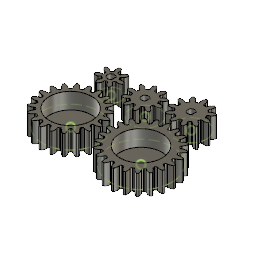
Telescope_Gears (Autodesk Fusion 360 design; units mm, degrees)
description: Spur Gear; Module: 2.0; Num Teeth: 20; Pressure Angle: 20.0; Backlash: 0.15 mm
description: Spur Gear; Module: 2.0; Num Teeth: 22; Pressure Angle: 20.0; Backlash: 0.15 mm
description: Spur Gear; Module: 2.0; Num Teeth: 11; Pressure Angle: 20.0; Backlash: 0.15 mm
description: Spur Gear; Module: 2.0; Num Teeth: 10; Pressure Angle: 20.0; Backlash: 0.15 mm
description: Spur Gear; Module: 2.0; Num Teeth: 7; Pressure Angle: 20.0; Backlash: 0.15 mm
Autodesk Fusion 360 part; units mm, degrees
(part 1 of 9)
sketch "Sketch1" plane through (0, 0, 0) normal (0, 0, 1) x (1, 0, 0) in component "Spur Gear (20 teeth) (1)"
  circle A0 centre (0, 0) radius 17.5492
  circle A1 centre (0, 0) radius 15
extrude "Extrude1" add sketch "Sketch1" along normal blind 11.5 makes body 1 in component "Spur Gear (20 teeth) (1)"
sketch "Sketch2" plane through (0, 0, 0) normal (0, 0, 1) x (1, 0, 0) in component "Spur Gear (20 teeth) (1)"
  spline S0 degree 5 poles (18.7151, -1.7185) (18.7245, -1.7194) (18.7433, -1.7209) (18.7715, -1.7223) (18.8091, -1.7228) (18.8563, -1.7215) (18.9035, -1.7188) (18.9507, -1.7153) (18.998, -1.7112) (19.0453, -1.7069) (19.0926, -1.7022) (19.1399, -1.697) (19.1872, -1.6913) (19.2346, -1.6849) (19.2819, -1.6778) (19.3293, -1.6701) (19.3766, -1.6618) (19.424, -1.6531) (19.4713, -1.644) (19.5186, -1.6345) (19.566, -1.6246) (19.6133, -1.6144) (19.6606, -1.6037) (19.7079, -1.5926) (19.7552, -1.581) (19.8025, -1.5691) (19.8498, -1.5568) (19.897, -1.5441) (19.9443, -1.531) (19.9915, -1.5176) (20.0387, -1.5039) (20.0858, -1.4898) (20.133, -1.4754) (20.1801, -1.4606) (20.2272, -1.4455) (20.2743, -1.43) (20.3213, -1.4143) (20.3683, -1.3982) (20.4153, -1.3818) (20.4623, -1.365) (20.5092, -1.348) (20.5561, -1.3307) (20.603, -1.313) (20.6498, -1.2951) (20.6966, -1.2768) (20.7434, -1.2583) (20.7901, -1.2394) (20.8368, -1.2203) (20.8835, -1.2009) (20.9301, -1.1812) (20.9767, -1.1612) (21.0233, -1.1409) (21.0698, -1.1204) (21.1162, -1.0995) (21.1627, -1.0784) (21.209, -1.0571) (21.2554, -1.0354) (21.3017, -1.0135) (21.3479, -0.9913) (21.3941, -0.9689) (21.4403, -0.9462) (21.4864, -0.9232) (21.5324, -0.8999) (21.5785, -0.8764) (21.6244, -0.8527) (21.6703, -0.8287) (21.7162, -0.8044) (21.762, -0.7799) (21.8078, -0.7551) (21.8535, -0.7301) (21.8991, -0.7049) (21.9356, -0.6845) (21.963, -0.669) (21.9812, -0.6587) (21.9903, -0.6535) knots 0 0 0 0 0 0 0.01428571 0.02857143 0.04285714 0.05714286 0.07142857 0.08571429 0.1 0.11428571 0.12857143 0.14285714 0.15714286 0.17142857 0.18571429 0.2 0.21428571 0.22857143 0.24285714 0.25714286 0.27142857 0.28571429 0.3 0.31428571 0.32857143 0.34285714 0.35714286 0.37142857 0.38571429 0.4 0.41428571 0.42857143 0.44285714 0.45714286 0.47142857 0.48571429 0.5 0.51428571 0.52857143 0.54285714 0.55714286 0.57142857 0.58571429 0.6 0.61428571 0.62857143 0.64285714 0.65714286 0.67142857 0.68571429 0.7 0.71428571 0.72857143 0.74285714 0.75714286 0.77142857 0.78571429 0.8 0.81428571 0.82857143 0.84285714 0.85714286 0.87142857 0.88571429 0.9 0.91428571 0.92857143 0.94285714 0.95714286 0.97142857 0.98571429 1 1 1 1 1 1
  spline S1 degree 5 poles (18.7151, 1.7185) (18.7245, 1.7194) (18.7433, 1.7209) (18.7715, 1.7223) (18.8091, 1.7228) (18.8563, 1.7215) (18.9035, 1.7188) (18.9507, 1.7153) (18.998, 1.7112) (19.0453, 1.7069) (19.0926, 1.7022) (19.1399, 1.697) (19.1872, 1.6913) (19.2346, 1.6849) (19.2819, 1.6778) (19.3293, 1.6701) (19.3766, 1.6618) (19.424, 1.6531) (19.4713, 1.644) (19.5186, 1.6345) (19.566, 1.6246) (19.6133, 1.6144) (19.6606, 1.6037) (19.7079, 1.5926) (19.7552, 1.581) (19.8025, 1.5691) (19.8498, 1.5568) (19.897, 1.5441) (19.9443, 1.531) (19.9915, 1.5176) (20.0387, 1.5039) (20.0858, 1.4898) (20.133, 1.4754) (20.1801, 1.4606) (20.2272, 1.4455) (20.2743, 1.43) (20.3213, 1.4143) (20.3683, 1.3982) (20.4153, 1.3818) (20.4623, 1.365) (20.5092, 1.348) (20.5561, 1.3307) (20.603, 1.313) (20.6498, 1.2951) (20.6966, 1.2768) (20.7434, 1.2583) (20.7901, 1.2394) (20.8368, 1.2203) (20.8835, 1.2009) (20.9301, 1.1812) (20.9767, 1.1612) (21.0233, 1.1409) (21.0698, 1.1204) (21.1162, 1.0995) (21.1627, 1.0784) (21.209, 1.0571) (21.2554, 1.0354) (21.3017, 1.0135) (21.3479, 0.9913) (21.3941, 0.9689) (21.4403, 0.9462) (21.4864, 0.9232) (21.5324, 0.8999) (21.5785, 0.8764) (21.6244, 0.8527) (21.6703, 0.8287) (21.7162, 0.8044) (21.762, 0.7799) (21.8078, 0.7551) (21.8535, 0.7301) (21.8991, 0.7049) (21.9356, 0.6845) (21.963, 0.669) (21.9812, 0.6587) (21.9903, 0.6535) knots 0 0 0 0 0 0 0.01428571 0.02857143 0.04285714 0.05714286 0.07142857 0.08571429 0.1 0.11428571 0.12857143 0.14285714 0.15714286 0.17142857 0.18571429 0.2 0.21428571 0.22857143 0.24285714 0.25714286 0.27142857 0.28571429 0.3 0.31428571 0.32857143 0.34285714 0.35714286 0.37142857 0.38571429 0.4 0.41428571 0.42857143 0.44285714 0.45714286 0.47142857 0.48571429 0.5 0.51428571 0.52857143 0.54285714 0.55714286 0.57142857 0.58571429 0.6 0.61428571 0.62857143 0.64285714 0.65714286 0.67142857 0.68571429 0.7 0.71428571 0.72857143 0.74285714 0.75714286 0.77142857 0.78571429 0.8 0.81428571 0.82857143 0.84285714 0.85714286 0.87142857 0.88571429 0.9 0.91428571 0.92857143 0.94285714 0.95714286 0.97142857 0.98571429 1 1 1 1 1 1
  arc A0 (21.9903, -0.6535) -> (21.9903, 0.6535) centre (0, 0) ccw
  line L0 (17.4657, -1.6047) -> (18.7151, -1.7185)
  line L1 (17.4657, 1.6047) -> (18.7151, 1.7185)
  line L2 (17.4657, -1.6047) -> (17.4657, 1.6047)
  point P0 (18.9453, -1.7156)
  point P1 (19.1773, -1.6924)
  point P2 (19.4104, -1.6555)
  point P3 (19.6442, -1.6073)
  point P4 (19.8786, -1.549)
  point P5 (20.1134, -1.4813)
  point P6 (20.3485, -1.4049)
  point P7 (20.5836, -1.3203)
  point P8 (20.8188, -1.2277)
  point P9 (21.0538, -1.1274)
  point P10 (21.2886, -1.0197)
  point P11 (21.523, -0.9047)
  point P12 (21.7569, -0.7826)
  point P13 (18.9453, 1.7156)
  point P14 (19.1773, 1.6924)
  point P15 (19.4104, 1.6555)
  point P16 (19.6442, 1.6073)
  point P17 (19.8786, 1.549)
  point P18 (20.1134, 1.4813)
  point P19 (20.3485, 1.4049)
  point P20 (20.5836, 1.3203)
  point P21 (20.8188, 1.2277)
  point P22 (21.0538, 1.1274)
  point P23 (21.2886, 1.0197)
  point P24 (21.523, 0.9047)
  point P25 (21.7569, 0.7826)
extrude "Extrude2" add sketch "Sketch2" along normal blind 11.5 bodies 1 in component "Spur Gear (20 teeth) (1)"
fillet "Fillet1" radius 0.9 2 edges at (17.4756, -1.6056, 5.75) (17.4756, 1.6056, 5.75) on bodies 1 in component "Spur Gear (20 teeth) (1)"
pattern_circular "C-Pattern1" count 20 over 360 about axis through (0, 0, 0) along (0, 0, 1) of "Extrude2", "Fillet1" in component "Spur Gear (20 teeth) (1)"
sketch "Sketch3" plane through (0, 0, 0) normal (0, 0, 1) x (1, 0, 0) in component "Spur Gear (20 teeth) (1)"
  circle A0 centre (0, 0) radius 20 construction
sketch "Sketch1 (2)" plane through (0, 0, 0) normal (0, 0, 1) x (1, 0, 0) in component "Spur Gear (22 teeth)"
  circle A0 centre (0, 0) radius 19.5492
  circle A1 centre (0, 0) radius 15
extrude "Extrude1'" add sketch "Sketch1 (2)" along normal blind 11.5 separate body makes body 2 in component "Spur Gear (22 teeth)"
sketch "Sketch2 (2)" plane through (0, 0, 0) normal (0, 0, 1) x (1, 0, 0) in component "Spur Gear (22 teeth)"
  spline S0 degree 5 poles (20.5993, -1.7469) (20.609, -1.7477) (20.6285, -1.7491) (20.6577, -1.7504) (20.6968, -1.7508) (20.7456, -1.7493) (20.7945, -1.7463) (20.8434, -1.7425) (20.8924, -1.7383) (20.9414, -1.7337) (20.9903, -1.7287) (21.0393, -1.7234) (21.0884, -1.7174) (21.1374, -1.7107) (21.1864, -1.7034) (21.2354, -1.6955) (21.2844, -1.6869) (21.3334, -1.678) (21.3825, -1.6686) (21.4315, -1.6589) (21.4805, -1.6487) (21.5294, -1.6382) (21.5784, -1.6273) (21.6274, -1.6159) (21.6763, -1.6041) (21.7253, -1.5919) (21.7742, -1.5794) (21.8231, -1.5664) (21.872, -1.5531) (21.9208, -1.5395) (21.9696, -1.5255) (22.0185, -1.5111) (22.0673, -1.4965) (22.116, -1.4814) (22.1648, -1.4661) (22.2135, -1.4504) (22.2622, -1.4343) (22.3109, -1.418) (22.3595, -1.4013) (22.4081, -1.3843) (22.4567, -1.3671) (22.5052, -1.3495) (22.5537, -1.3316) (22.6022, -1.3134) (22.6507, -1.2949) (22.6991, -1.2761) (22.7475, -1.257) (22.7958, -1.2376) (22.8441, -1.218) (22.8924, -1.198) (22.9406, -1.1778) (22.9888, -1.1573) (23.037, -1.1365) (23.0851, -1.1154) (23.1332, -1.0941) (23.1812, -1.0724) (23.2292, -1.0506) (23.2772, -1.0284) (23.3251, -1.006) (23.3729, -0.9833) (23.4207, -0.9604) (23.4685, -0.9372) (23.5162, -0.9137) (23.5639, -0.89) (23.6115, -0.866) (23.6591, -0.8417) (23.7067, -0.8173) (23.7541, -0.7925) (23.8016, -0.7675) (23.849, -0.7423) (23.8963, -0.7168) (23.9341, -0.6962) (23.9625, -0.6807) (23.9813, -0.6702) (23.9908, -0.665) knots 0 0 0 0 0 0 0.01428571 0.02857143 0.04285714 0.05714286 0.07142857 0.08571429 0.1 0.11428571 0.12857143 0.14285714 0.15714286 0.17142857 0.18571429 0.2 0.21428571 0.22857143 0.24285714 0.25714286 0.27142857 0.28571429 0.3 0.31428571 0.32857143 0.34285714 0.35714286 0.37142857 0.38571429 0.4 0.41428571 0.42857143 0.44285714 0.45714286 0.47142857 0.48571429 0.5 0.51428571 0.52857143 0.54285714 0.55714286 0.57142857 0.58571429 0.6 0.61428571 0.62857143 0.64285714 0.65714286 0.67142857 0.68571429 0.7 0.71428571 0.72857143 0.74285714 0.75714286 0.77142857 0.78571429 0.8 0.81428571 0.82857143 0.84285714 0.85714286 0.87142857 0.88571429 0.9 0.91428571 0.92857143 0.94285714 0.95714286 0.97142857 0.98571429 1 1 1 1 1 1
  spline S1 degree 5 poles (20.5993, 1.7469) (20.609, 1.7477) (20.6285, 1.7491) (20.6577, 1.7504) (20.6968, 1.7508) (20.7456, 1.7493) (20.7945, 1.7463) (20.8434, 1.7425) (20.8924, 1.7383) (20.9414, 1.7337) (20.9903, 1.7287) (21.0393, 1.7234) (21.0884, 1.7174) (21.1374, 1.7107) (21.1864, 1.7034) (21.2354, 1.6955) (21.2844, 1.6869) (21.3334, 1.678) (21.3825, 1.6686) (21.4315, 1.6589) (21.4805, 1.6487) (21.5294, 1.6382) (21.5784, 1.6273) (21.6274, 1.6159) (21.6763, 1.6041) (21.7253, 1.5919) (21.7742, 1.5794) (21.8231, 1.5664) (21.872, 1.5531) (21.9208, 1.5395) (21.9696, 1.5255) (22.0185, 1.5111) (22.0673, 1.4965) (22.116, 1.4814) (22.1648, 1.4661) (22.2135, 1.4504) (22.2622, 1.4343) (22.3109, 1.418) (22.3595, 1.4013) (22.4081, 1.3843) (22.4567, 1.3671) (22.5052, 1.3495) (22.5537, 1.3316) (22.6022, 1.3134) (22.6507, 1.2949) (22.6991, 1.2761) (22.7475, 1.257) (22.7958, 1.2376) (22.8441, 1.218) (22.8924, 1.198) (22.9406, 1.1778) (22.9888, 1.1573) (23.037, 1.1365) (23.0851, 1.1154) (23.1332, 1.0941) (23.1812, 1.0724) (23.2292, 1.0506) (23.2772, 1.0284) (23.3251, 1.006) (23.3729, 0.9833) (23.4207, 0.9604) (23.4685, 0.9372) (23.5162, 0.9137) (23.5639, 0.89) (23.6115, 0.866) (23.6591, 0.8417) (23.7067, 0.8173) (23.7541, 0.7925) (23.8016, 0.7675) (23.849, 0.7423) (23.8963, 0.7168) (23.9341, 0.6962) (23.9625, 0.6807) (23.9813, 0.6702) (23.9908, 0.665) knots 0 0 0 0 0 0 0.01428571 0.02857143 0.04285714 0.05714286 0.07142857 0.08571429 0.1 0.11428571 0.12857143 0.14285714 0.15714286 0.17142857 0.18571429 0.2 0.21428571 0.22857143 0.24285714 0.25714286 0.27142857 0.28571429 0.3 0.31428571 0.32857143 0.34285714 0.35714286 0.37142857 0.38571429 0.4 0.41428571 0.42857143 0.44285714 0.45714286 0.47142857 0.48571429 0.5 0.51428571 0.52857143 0.54285714 0.55714286 0.57142857 0.58571429 0.6 0.61428571 0.62857143 0.64285714 0.65714286 0.67142857 0.68571429 0.7 0.71428571 0.72857143 0.74285714 0.75714286 0.77142857 0.78571429 0.8 0.81428571 0.82857143 0.84285714 0.85714286 0.87142857 0.88571429 0.9 0.91428571 0.92857143 0.94285714 0.95714286 0.97142857 0.98571429 1 1 1 1 1 1
  arc A0 (23.9908, -0.665) -> (23.9908, 0.665) centre (0, 0) ccw
  line L0 (19.4693, -1.6519) -> (20.5993, -1.7469)
  line L1 (19.4693, 1.6519) -> (20.5993, 1.7469)
  line L2 (19.4693, -1.6519) -> (19.4693, 1.6519)
  point P0 (20.8381, -1.7429)
  point P1 (21.0786, -1.7185)
  point P2 (21.32, -1.6804)
  point P3 (21.5622, -1.6309)
  point P4 (21.8048, -1.5712)
  point P5 (22.0479, -1.5022)
  point P6 (22.2911, -1.4246)
  point P7 (22.5345, -1.3386)
  point P8 (22.7779, -1.2448)
  point P9 (23.0211, -1.1433)
  point P10 (23.2641, -1.0344)
  point P11 (23.5068, -0.9183)
  point P12 (23.7491, -0.7951)
  point P13 (20.8381, 1.7429)
  point P14 (21.0786, 1.7185)
  point P15 (21.32, 1.6804)
  point P16 (21.5622, 1.6309)
  point P17 (21.8048, 1.5712)
  point P18 (22.0479, 1.5022)
  point P19 (22.2911, 1.4246)
  point P20 (22.5345, 1.3386)
  point P21 (22.7779, 1.2448)
  point P22 (23.0211, 1.1433)
  point P23 (23.2641, 1.0344)
  point P24 (23.5068, 0.9183)
  point P25 (23.7491, 0.7951)
extrude "Extrude2'" add sketch "Sketch2 (2)" along normal blind 11.5 bodies 2 in component "Spur Gear (22 teeth)"
fillet "Fillet1'" radius 1 2 edges at (19.4792, -1.6527, 5.75) (19.4792, 1.6527, 5.75) on bodies 2 in component "Spur Gear (22 teeth)"
pattern_circular "C-Pattern1'" count 22 over 360 about axis through (0, 0, 0) along (0, 0, 1) of "Extrude2'", "Fillet1'" in component "Spur Gear (22 teeth)"
sketch "Sketch3 (2)" plane through (0, 0, 0) normal (0, 0, 1) x (1, 0, 0) in component "Spur Gear (22 teeth)"
  circle A0 centre (0, 0) radius 22 construction
sketch "Sketch1 (3)" plane through (0, 0, 0) normal (0, 0, 1) x (1, 0, 0) in component "Spur Gear (11 teeth)"
  circle A0 centre (0, 0) radius 8.5492
  circle A1 centre (0, 0) radius 2.5
extrude "Extrude1''" add sketch "Sketch1 (3)" along normal blind 11.5 separate body makes body 3 in component "Spur Gear (11 teeth)"
sketch "Sketch2 (3)" plane through (0, 0, 0) normal (0, 0, 1) x (1, 0, 0) in component "Spur Gear (11 teeth)"
  spline S0 degree 5 poles (10.2138, -1.5886) (10.2216, -1.5898) (10.2373, -1.5919) (10.2609, -1.5944) (10.2925, -1.5962) (10.3321, -1.5965) (10.3719, -1.5954) (10.4117, -1.5933) (10.4517, -1.5907) (10.4917, -1.5878) (10.5317, -1.5846) (10.5717, -1.5809) (10.6118, -1.5765) (10.6519, -1.5714) (10.6921, -1.5656) (10.7323, -1.5592) (10.7726, -1.5521) (10.8128, -1.5446) (10.8531, -1.5367) (10.8933, -1.5283) (10.9336, -1.5196) (10.9739, -1.5104) (11.0141, -1.5007) (11.0544, -1.4906) (11.0947, -1.4801) (11.135, -1.4691) (11.1752, -1.4577) (11.2155, -1.4459) (11.2557, -1.4337) (11.2959, -1.4211) (11.3362, -1.4082) (11.3763, -1.3948) (11.4165, -1.3811) (11.4567, -1.367) (11.4968, -1.3526) (11.5369, -1.3378) (11.577, -1.3226) (11.617, -1.307) (11.657, -1.2912) (11.697, -1.2749) (11.7369, -1.2583) (11.7769, -1.2414) (11.8167, -1.2242) (11.8566, -1.2066) (11.8963, -1.1887) (11.9361, -1.1704) (11.9758, -1.1518) (12.0154, -1.1329) (12.0551, -1.1137) (12.0946, -1.0941) (12.1341, -1.0743) (12.1736, -1.0541) (12.213, -1.0336) (12.2524, -1.0128) (12.2916, -0.9917) (12.3309, -0.9703) (12.3701, -0.9486) (12.4092, -0.9265) (12.4482, -0.9042) (12.4872, -0.8816) (12.5262, -0.8587) (12.565, -0.8355) (12.6038, -0.812) (12.6426, -0.7882) (12.6812, -0.7641) (12.7198, -0.7397) (12.7584, -0.715) (12.7968, -0.6901) (12.8352, -0.6649) (12.8735, -0.6393) (12.9117, -0.6136) (12.9422, -0.5927) (12.9651, -0.5769) (12.9803, -0.5664) (12.9879, -0.5611) knots 0 0 0 0 0 0 0.01428571 0.02857143 0.04285714 0.05714286 0.07142857 0.08571429 0.1 0.11428571 0.12857143 0.14285714 0.15714286 0.17142857 0.18571429 0.2 0.21428571 0.22857143 0.24285714 0.25714286 0.27142857 0.28571429 0.3 0.31428571 0.32857143 0.34285714 0.35714286 0.37142857 0.38571429 0.4 0.41428571 0.42857143 0.44285714 0.45714286 0.47142857 0.48571429 0.5 0.51428571 0.52857143 0.54285714 0.55714286 0.57142857 0.58571429 0.6 0.61428571 0.62857143 0.64285714 0.65714286 0.67142857 0.68571429 0.7 0.71428571 0.72857143 0.74285714 0.75714286 0.77142857 0.78571429 0.8 0.81428571 0.82857143 0.84285714 0.85714286 0.87142857 0.88571429 0.9 0.91428571 0.92857143 0.94285714 0.95714286 0.97142857 0.98571429 1 1 1 1 1 1
  spline S1 degree 5 poles (10.2138, 1.5886) (10.2216, 1.5898) (10.2373, 1.5919) (10.2609, 1.5944) (10.2925, 1.5962) (10.3321, 1.5965) (10.3719, 1.5954) (10.4117, 1.5933) (10.4517, 1.5907) (10.4917, 1.5878) (10.5317, 1.5846) (10.5717, 1.5809) (10.6118, 1.5765) (10.6519, 1.5714) (10.6921, 1.5656) (10.7323, 1.5592) (10.7726, 1.5521) (10.8128, 1.5446) (10.8531, 1.5367) (10.8933, 1.5283) (10.9336, 1.5196) (10.9739, 1.5104) (11.0141, 1.5007) (11.0544, 1.4906) (11.0947, 1.4801) (11.135, 1.4691) (11.1752, 1.4577) (11.2155, 1.4459) (11.2557, 1.4337) (11.2959, 1.4211) (11.3362, 1.4082) (11.3763, 1.3948) (11.4165, 1.3811) (11.4567, 1.367) (11.4968, 1.3526) (11.5369, 1.3378) (11.577, 1.3226) (11.617, 1.307) (11.657, 1.2912) (11.697, 1.2749) (11.7369, 1.2583) (11.7769, 1.2414) (11.8167, 1.2242) (11.8566, 1.2066) (11.8963, 1.1887) (11.9361, 1.1704) (11.9758, 1.1518) (12.0154, 1.1329) (12.0551, 1.1137) (12.0946, 1.0941) (12.1341, 1.0743) (12.1736, 1.0541) (12.213, 1.0336) (12.2524, 1.0128) (12.2916, 0.9917) (12.3309, 0.9703) (12.3701, 0.9486) (12.4092, 0.9265) (12.4482, 0.9042) (12.4872, 0.8816) (12.5262, 0.8587) (12.565, 0.8355) (12.6038, 0.812) (12.6426, 0.7882) (12.6812, 0.7641) (12.7198, 0.7397) (12.7584, 0.715) (12.7968, 0.6901) (12.8352, 0.6649) (12.8735, 0.6393) (12.9117, 0.6136) (12.9422, 0.5927) (12.9651, 0.5769) (12.9803, 0.5664) (12.9879, 0.5611) knots 0 0 0 0 0 0 0.01428571 0.02857143 0.04285714 0.05714286 0.07142857 0.08571429 0.1 0.11428571 0.12857143 0.14285714 0.15714286 0.17142857 0.18571429 0.2 0.21428571 0.22857143 0.24285714 0.25714286 0.27142857 0.28571429 0.3 0.31428571 0.32857143 0.34285714 0.35714286 0.37142857 0.38571429 0.4 0.41428571 0.42857143 0.44285714 0.45714286 0.47142857 0.48571429 0.5 0.51428571 0.52857143 0.54285714 0.55714286 0.57142857 0.58571429 0.6 0.61428571 0.62857143 0.64285714 0.65714286 0.67142857 0.68571429 0.7 0.71428571 0.72857143 0.74285714 0.75714286 0.77142857 0.78571429 0.8 0.81428571 0.82857143 0.84285714 0.85714286 0.87142857 0.88571429 0.9 0.91428571 0.92857143 0.94285714 0.95714286 0.97142857 0.98571429 1 1 1 1 1 1
  arc A0 (12.9879, -0.5611) -> (12.9879, 0.5611) centre (0, 0) ccw
  line L0 (8.4378, -1.3139) -> (10.2138, -1.5886)
  line L1 (8.4378, 1.3139) -> (10.2138, 1.5886)
  line L2 (8.4378, -1.3139) -> (8.4378, 1.3139)
  point P0 (10.4056, -1.5935)
  point P1 (10.6003, -1.5776)
  point P2 (10.797, -1.5475)
  point P3 (10.995, -1.5052)
  point P4 (11.194, -1.4521)
  point P5 (11.3937, -1.3888)
  point P6 (11.5939, -1.316)
  point P7 (11.7942, -1.2339)
  point P8 (11.9945, -1.1429)
  point P9 (12.1945, -1.0432)
  point P10 (12.3941, -0.935)
  point P11 (12.5929, -0.8185)
  point P12 (12.791, -0.6938)
  point P13 (10.4056, 1.5935)
  point P14 (10.6003, 1.5776)
  point P15 (10.797, 1.5475)
  point P16 (10.995, 1.5052)
  point P17 (11.194, 1.4521)
  point P18 (11.3937, 1.3888)
  point P19 (11.5939, 1.316)
  point P20 (11.7942, 1.2339)
  point P21 (11.9945, 1.1429)
  point P22 (12.1945, 1.0432)
  point P23 (12.3941, 0.935)
  point P24 (12.5929, 0.8185)
  point P25 (12.791, 0.6938)
extrude "Extrude2''" add sketch "Sketch2 (3)" along normal blind 11.5 bodies 3 in component "Spur Gear (11 teeth)"
fillet "Fillet1''" radius 0.5 2 edges at (8.4474, -1.3154, 5.75) (8.4474, 1.3154, 5.75) on bodies 3 in component "Spur Gear (11 teeth)"
pattern_circular "C-Pattern1''" count 11 over 360 about axis through (0, 0, 0) along (0, 0, 1) of "Extrude2''", "Fillet1''" in component "Spur Gear (11 teeth)"
sketch "Sketch3 (3)" plane through (0, 0, 0) normal (0, 0, 1) x (1, 0, 0) in component "Spur Gear (11 teeth)"
  circle A0 centre (0, 0) radius 11 construction
sketch "Sketch1 (4)" plane through (0, 0, 0) normal (0, 0, 1) x (1, 0, 0) in component "Spur Gear (10 teeth)"
  circle A0 centre (0, 0) radius 7.5492
  circle A1 centre (0, 0) radius 2.5
extrude "Extrude1'''" add sketch "Sketch1 (4)" along normal blind 11.5 separate body makes body 4 in component "Spur Gear (10 teeth)"
sketch "Sketch2 (4)" plane through (0, 0, 0) normal (0, 0, 1) x (1, 0, 0) in component "Spur Gear (10 teeth)"
  spline S0 degree 5 poles (9.2643, -1.5734) (9.2719, -1.5747) (9.2872, -1.5771) (9.3103, -1.5797) (9.3412, -1.5819) (9.38, -1.5824) (9.419, -1.5816) (9.4582, -1.5798) (9.4973, -1.5775) (9.5366, -1.5749) (9.5758, -1.5719) (9.6151, -1.5684) (9.6545, -1.5643) (9.6939, -1.5594) (9.7333, -1.5538) (9.7728, -1.5475) (9.8124, -1.5407) (9.8519, -1.5333) (9.8915, -1.5255) (9.931, -1.5173) (9.9706, -1.5087) (10.0102, -1.4996) (10.0498, -1.4901) (10.0894, -1.4801) (10.129, -1.4697) (10.1686, -1.4587) (10.2082, -1.4474) (10.2477, -1.4356) (10.2873, -1.4235) (10.3269, -1.411) (10.3664, -1.398) (10.4059, -1.3847) (10.4454, -1.371) (10.4849, -1.3569) (10.5243, -1.3424) (10.5638, -1.3276) (10.6032, -1.3124) (10.6425, -1.2968) (10.6819, -1.2808) (10.7212, -1.2645) (10.7604, -1.2479) (10.7997, -1.2308) (10.8388, -1.2135) (10.878, -1.1958) (10.9171, -1.1777) (10.9561, -1.1593) (10.9952, -1.1406) (11.0341, -1.1215) (11.073, -1.1022) (11.1119, -1.0824) (11.1507, -1.0624) (11.1894, -1.042) (11.2281, -1.0213) (11.2668, -1.0003) (11.3054, -0.9789) (11.3439, -0.9573) (11.3823, -0.9353) (11.4207, -0.913) (11.459, -0.8905) (11.4973, -0.8676) (11.5355, -0.8443) (11.5736, -0.8208) (11.6116, -0.797) (11.6496, -0.7729) (11.6875, -0.7485) (11.7253, -0.7238) (11.763, -0.6988) (11.8007, -0.6735) (11.8383, -0.6479) (11.8758, -0.622) (11.9132, -0.5958) (11.943, -0.5746) (11.9654, -0.5586) (11.9803, -0.5479) (11.9877, -0.5425) knots 0 0 0 0 0 0 0.01428571 0.02857143 0.04285714 0.05714286 0.07142857 0.08571429 0.1 0.11428571 0.12857143 0.14285714 0.15714286 0.17142857 0.18571429 0.2 0.21428571 0.22857143 0.24285714 0.25714286 0.27142857 0.28571429 0.3 0.31428571 0.32857143 0.34285714 0.35714286 0.37142857 0.38571429 0.4 0.41428571 0.42857143 0.44285714 0.45714286 0.47142857 0.48571429 0.5 0.51428571 0.52857143 0.54285714 0.55714286 0.57142857 0.58571429 0.6 0.61428571 0.62857143 0.64285714 0.65714286 0.67142857 0.68571429 0.7 0.71428571 0.72857143 0.74285714 0.75714286 0.77142857 0.78571429 0.8 0.81428571 0.82857143 0.84285714 0.85714286 0.87142857 0.88571429 0.9 0.91428571 0.92857143 0.94285714 0.95714286 0.97142857 0.98571429 1 1 1 1 1 1
  spline S1 degree 5 poles (9.2643, 1.5734) (9.2719, 1.5747) (9.2872, 1.5771) (9.3103, 1.5797) (9.3412, 1.5819) (9.38, 1.5824) (9.419, 1.5816) (9.4582, 1.5798) (9.4973, 1.5775) (9.5366, 1.5749) (9.5758, 1.5719) (9.6151, 1.5684) (9.6545, 1.5643) (9.6939, 1.5594) (9.7333, 1.5538) (9.7728, 1.5475) (9.8124, 1.5407) (9.8519, 1.5333) (9.8915, 1.5255) (9.931, 1.5173) (9.9706, 1.5087) (10.0102, 1.4996) (10.0498, 1.4901) (10.0894, 1.4801) (10.129, 1.4697) (10.1686, 1.4587) (10.2082, 1.4474) (10.2477, 1.4356) (10.2873, 1.4235) (10.3269, 1.411) (10.3664, 1.398) (10.4059, 1.3847) (10.4454, 1.371) (10.4849, 1.3569) (10.5243, 1.3424) (10.5638, 1.3276) (10.6032, 1.3124) (10.6425, 1.2968) (10.6819, 1.2808) (10.7212, 1.2645) (10.7604, 1.2479) (10.7997, 1.2308) (10.8388, 1.2135) (10.878, 1.1958) (10.9171, 1.1777) (10.9561, 1.1593) (10.9952, 1.1406) (11.0341, 1.1215) (11.073, 1.1022) (11.1119, 1.0824) (11.1507, 1.0624) (11.1894, 1.042) (11.2281, 1.0213) (11.2668, 1.0003) (11.3054, 0.9789) (11.3439, 0.9573) (11.3823, 0.9353) (11.4207, 0.913) (11.459, 0.8905) (11.4973, 0.8676) (11.5355, 0.8443) (11.5736, 0.8208) (11.6116, 0.797) (11.6496, 0.7729) (11.6875, 0.7485) (11.7253, 0.7238) (11.763, 0.6988) (11.8007, 0.6735) (11.8383, 0.6479) (11.8758, 0.622) (11.9132, 0.5958) (11.943, 0.5746) (11.9654, 0.5586) (11.9803, 0.5479) (11.9877, 0.5425) knots 0 0 0 0 0 0 0.01428571 0.02857143 0.04285714 0.05714286 0.07142857 0.08571429 0.1 0.11428571 0.12857143 0.14285714 0.15714286 0.17142857 0.18571429 0.2 0.21428571 0.22857143 0.24285714 0.25714286 0.27142857 0.28571429 0.3 0.31428571 0.32857143 0.34285714 0.35714286 0.37142857 0.38571429 0.4 0.41428571 0.42857143 0.44285714 0.45714286 0.47142857 0.48571429 0.5 0.51428571 0.52857143 0.54285714 0.55714286 0.57142857 0.58571429 0.6 0.61428571 0.62857143 0.64285714 0.65714286 0.67142857 0.68571429 0.7 0.71428571 0.72857143 0.74285714 0.75714286 0.77142857 0.78571429 0.8 0.81428571 0.82857143 0.84285714 0.85714286 0.87142857 0.88571429 0.9 0.91428571 0.92857143 0.94285714 0.95714286 0.97142857 0.98571429 1 1 1 1 1 1
  arc A0 (11.9877, -0.5425) -> (11.9877, 0.5425) centre (0, 0) ccw
  line L0 (7.4328, -1.264) -> (9.2643, -1.5734)
  line L1 (7.4328, 1.264) -> (9.2643, 1.5734)
  line L2 (7.4328, -1.264) -> (7.4328, 1.264)
  point P0 (9.4517, -1.58)
  point P1 (9.6426, -1.5654)
  point P2 (9.8355, -1.5363)
  point P3 (10.0299, -1.4948)
  point P4 (10.2254, -1.4422)
  point P5 (10.4217, -1.3792)
  point P6 (10.6184, -1.3063)
  point P7 (10.8154, -1.2238)
  point P8 (11.0123, -1.1322)
  point P9 (11.2089, -1.0316)
  point P10 (11.405, -0.9221)
  point P11 (11.6003, -0.8041)
  point P12 (11.7946, -0.6775)
  point P13 (9.4517, 1.58)
  point P14 (9.6426, 1.5654)
  point P15 (9.8355, 1.5363)
  point P16 (10.0299, 1.4948)
  point P17 (10.2254, 1.4422)
  point P18 (10.4217, 1.3792)
  point P19 (10.6184, 1.3063)
  point P20 (10.8154, 1.2238)
  point P21 (11.0123, 1.1322)
  point P22 (11.2089, 1.0316)
  point P23 (11.405, 0.9221)
  point P24 (11.6003, 0.8041)
  point P25 (11.7946, 0.6775)
extrude "Extrude2'''" add sketch "Sketch2 (4)" along normal blind 11.5 bodies 4 in component "Spur Gear (10 teeth)"
fillet "Fillet1'''" radius 0.5 2 edges at (7.4423, -1.2657, 5.75) (7.4423, 1.2657, 5.75) on bodies 4 in component "Spur Gear (10 teeth)"
pattern_circular "C-Pattern1'''" count 10 over 360 about axis through (0, 0, 0) along (0, 0, 1) of "Extrude2'''", "Fillet1'''" in component "Spur Gear (10 teeth)"
sketch "Sketch3 (4)" plane through (0, 0, 0) normal (0, 0, 1) x (1, 0, 0) in component "Spur Gear (10 teeth)"
  circle A0 centre (0, 0) radius 10 construction
sketch "Sketch1 (5)" plane through (0, 0, 0) normal (0, 0, 1) x (1, 0, 0) in component "Spur Gear (7 teeth)"
  circle A0 centre (0, 0) radius 4.5492
  circle A1 centre (0, 0) radius 2.5
extrude "Extrude1''''" add sketch "Sketch1 (5)" along normal blind 11.5 separate body makes body 5 in component "Spur Gear (7 teeth)"
sketch "Sketch2 (5)" plane through (0, 0, 0) normal (0, 0, 1) x (1, 0, 0) in component "Spur Gear (7 teeth)"
  spline S0 degree 5 poles (6.3987, -1.5249) (6.4058, -1.5266) (6.42, -1.5296) (6.4416, -1.5334) (6.4705, -1.5368) (6.507, -1.5389) (6.5438, -1.5394) (6.5808, -1.5389) (6.6179, -1.5378) (6.6551, -1.5364) (6.6923, -1.5346) (6.7296, -1.5321) (6.767, -1.529) (6.8045, -1.5251) (6.8421, -1.5203) (6.8797, -1.5148) (6.9174, -1.5087) (6.9552, -1.502) (6.993, -1.4948) (7.0308, -1.4872) (7.0686, -1.4791) (7.1065, -1.4705) (7.1444, -1.4613) (7.1823, -1.4516) (7.2202, -1.4414) (7.2581, -1.4307) (7.296, -1.4195) (7.334, -1.4078) (7.3719, -1.3957) (7.4098, -1.3831) (7.4477, -1.3701) (7.4856, -1.3567) (7.5234, -1.3428) (7.5613, -1.3284) (7.5991, -1.3136) (7.6369, -1.2984) (7.6746, -1.2827) (7.7123, -1.2666) (7.75, -1.2502) (7.7876, -1.2333) (7.8252, -1.2159) (7.8627, -1.1982) (7.9002, -1.1801) (7.9377, -1.1616) (7.975, -1.1426) (8.0124, -1.1233) (8.0496, -1.1036) (8.0868, -1.0835) (8.1239, -1.063) (8.161, -1.0421) (8.198, -1.0209) (8.2349, -0.9993) (8.2717, -0.9772) (8.3085, -0.9549) (8.3451, -0.9321) (8.3817, -0.909) (8.4182, -0.8855) (8.4546, -0.8617) (8.4909, -0.8374) (8.5271, -0.8129) (8.5632, -0.7879) (8.5992, -0.7627) (8.6352, -0.737) (8.671, -0.711) (8.7067, -0.6847) (8.7423, -0.658) (8.7778, -0.631) (8.8131, -0.6036) (8.8484, -0.5759) (8.8835, -0.5478) (8.9185, -0.5194) (8.9464, -0.4965) (8.9673, -0.4791) (8.9812, -0.4674) (8.9882, -0.4616) knots 0 0 0 0 0 0 0.01428571 0.02857143 0.04285714 0.05714286 0.07142857 0.08571429 0.1 0.11428571 0.12857143 0.14285714 0.15714286 0.17142857 0.18571429 0.2 0.21428571 0.22857143 0.24285714 0.25714286 0.27142857 0.28571429 0.3 0.31428571 0.32857143 0.34285714 0.35714286 0.37142857 0.38571429 0.4 0.41428571 0.42857143 0.44285714 0.45714286 0.47142857 0.48571429 0.5 0.51428571 0.52857143 0.54285714 0.55714286 0.57142857 0.58571429 0.6 0.61428571 0.62857143 0.64285714 0.65714286 0.67142857 0.68571429 0.7 0.71428571 0.72857143 0.74285714 0.75714286 0.77142857 0.78571429 0.8 0.81428571 0.82857143 0.84285714 0.85714286 0.87142857 0.88571429 0.9 0.91428571 0.92857143 0.94285714 0.95714286 0.97142857 0.98571429 1 1 1 1 1 1
  spline S1 degree 5 poles (6.3987, 1.5249) (6.4058, 1.5266) (6.42, 1.5296) (6.4416, 1.5334) (6.4705, 1.5368) (6.507, 1.5389) (6.5438, 1.5394) (6.5808, 1.5389) (6.6179, 1.5378) (6.6551, 1.5364) (6.6923, 1.5346) (6.7296, 1.5321) (6.767, 1.529) (6.8045, 1.5251) (6.8421, 1.5203) (6.8797, 1.5148) (6.9174, 1.5087) (6.9552, 1.502) (6.993, 1.4948) (7.0308, 1.4872) (7.0686, 1.4791) (7.1065, 1.4705) (7.1444, 1.4613) (7.1823, 1.4516) (7.2202, 1.4414) (7.2581, 1.4307) (7.296, 1.4195) (7.334, 1.4078) (7.3719, 1.3957) (7.4098, 1.3831) (7.4477, 1.3701) (7.4856, 1.3567) (7.5234, 1.3428) (7.5613, 1.3284) (7.5991, 1.3136) (7.6369, 1.2984) (7.6746, 1.2827) (7.7123, 1.2666) (7.75, 1.2502) (7.7876, 1.2333) (7.8252, 1.2159) (7.8627, 1.1982) (7.9002, 1.1801) (7.9377, 1.1616) (7.975, 1.1426) (8.0124, 1.1233) (8.0496, 1.1036) (8.0868, 1.0835) (8.1239, 1.063) (8.161, 1.0421) (8.198, 1.0209) (8.2349, 0.9993) (8.2717, 0.9772) (8.3085, 0.9549) (8.3451, 0.9321) (8.3817, 0.909) (8.4182, 0.8855) (8.4546, 0.8617) (8.4909, 0.8374) (8.5271, 0.8129) (8.5632, 0.7879) (8.5992, 0.7627) (8.6352, 0.737) (8.671, 0.711) (8.7067, 0.6847) (8.7423, 0.658) (8.7778, 0.631) (8.8131, 0.6036) (8.8484, 0.5759) (8.8835, 0.5478) (8.9185, 0.5194) (8.9464, 0.4965) (8.9673, 0.4791) (8.9812, 0.4674) (8.9882, 0.4616) knots 0 0 0 0 0 0 0.01428571 0.02857143 0.04285714 0.05714286 0.07142857 0.08571429 0.1 0.11428571 0.12857143 0.14285714 0.15714286 0.17142857 0.18571429 0.2 0.21428571 0.22857143 0.24285714 0.25714286 0.27142857 0.28571429 0.3 0.31428571 0.32857143 0.34285714 0.35714286 0.37142857 0.38571429 0.4 0.41428571 0.42857143 0.44285714 0.45714286 0.47142857 0.48571429 0.5 0.51428571 0.52857143 0.54285714 0.55714286 0.57142857 0.58571429 0.6 0.61428571 0.62857143 0.64285714 0.65714286 0.67142857 0.68571429 0.7 0.71428571 0.72857143 0.74285714 0.75714286 0.77142857 0.78571429 0.8 0.81428571 0.82857143 0.84285714 0.85714286 0.87142857 0.88571429 0.9 0.91428571 0.92857143 0.94285714 0.95714286 0.97142857 0.98571429 1 1 1 1 1 1
  arc A0 (8.9882, -0.4616) -> (8.9882, 0.4616) centre (0, 0) ccw
  line L0 (4.4155, -1.0546) -> (6.3987, -1.5249)
  line L1 (4.4155, 1.0546) -> (6.3987, 1.5249)
  line L2 (4.4155, -1.0546) -> (4.4155, 1.0546)
  point P0 (6.5731, -1.5389)
  point P1 (6.7527, -1.5301)
  point P2 (6.9354, -1.5055)
  point P3 (7.1203, -1.4671)
  point P4 (7.3069, -1.4161)
  point P5 (7.4947, -1.3532)
  point P6 (7.6832, -1.279)
  point P7 (7.8719, -1.1937)
  point P8 (8.0606, -1.0976)
  point P9 (8.2486, -0.991)
  point P10 (8.4358, -0.8739)
  point P11 (8.6217, -0.7466)
  point P12 (8.806, -0.6091)
  point P13 (6.5731, 1.5389)
  point P14 (6.7527, 1.5301)
  point P15 (6.9354, 1.5055)
  point P16 (7.1203, 1.4671)
  point P17 (7.3069, 1.4161)
  point P18 (7.4947, 1.3532)
  point P19 (7.6832, 1.279)
  point P20 (7.8719, 1.1937)
  point P21 (8.0606, 1.0976)
  point P22 (8.2486, 0.991)
  point P23 (8.4358, 0.8739)
  point P24 (8.6217, 0.7466)
  point P25 (8.806, 0.6091)
extrude "Extrude2''''" add sketch "Sketch2 (5)" along normal blind 11.5 bodies 5 in component "Spur Gear (7 teeth)"
fillet "Fillet1''''" radius 0.5 2 edges at (4.4248, -1.0568, 5.75) (4.4248, 1.0568, 5.75) on bodies 5 in component "Spur Gear (7 teeth)"
pattern_circular "C-Pattern1''''" count 7 over 360 about axis through (0, 0, 0) along (0, 0, 1) of "Extrude2''''", "Fillet1''''" in component "Spur Gear (7 teeth)"
sketch "Sketch3 (5)" plane through (0, 0, 0) normal (0, 0, 1) x (1, 0, 0) in component "Spur Gear (7 teeth)"
  circle A0 centre (0, 0) radius 7 construction
sketch "Sketch3 (6)" plane through (0, 0, 11.1684) normal (0, 0, 1) x (-1, 0, 0)
  arc A0 (-19.4404, -30.8508) -> (-19.83, -32.0501) centre (-12.4806, -33.7751) ccw
  arc A1 (-20.4001, -32.4289) -> (-19.83, -32.0501) centre (-20.3168, -31.9359) ccw
  line L0 (-20.4001, -32.4289) -> (-21.7448, -32.2017)
  spline S0 degree 5 poles (-21.7448, -32.2017) (-21.7525, -32.2004) (-21.7678, -32.1981) (-21.7909, -32.1954) (-21.8218, -32.1933) (-21.8606, -32.1927) (-21.8996, -32.1936) (-21.9387, -32.1954) (-21.9779, -32.1976) (-22.0171, -32.2003) (-22.0564, -32.2033) (-22.0957, -32.2067) (-22.1351, -32.2109) (-22.1745, -32.2157) (-22.2139, -32.2213) (-22.2534, -32.2276) (-22.2929, -32.2345) (-22.3325, -32.2418) (-22.372, -32.2496) (-22.4116, -32.2578) (-22.4512, -32.2664) (-22.4908, -32.2755) (-22.5304, -32.285) (-22.5699, -32.295) (-22.6095, -32.3055) (-22.6491, -32.3164) (-22.6887, -32.3277) (-22.7283, -32.3395) (-22.7679, -32.3517) (-22.8074, -32.3642) (-22.847, -32.3771) (-22.8865, -32.3904) (-22.926, -32.4041) (-22.9654, -32.4182) (-23.0049, -32.4327) (-23.0443, -32.4476) (-23.0837, -32.4628) (-23.1231, -32.4784) (-23.1624, -32.4943) (-23.2017, -32.5106) (-23.241, -32.5273) (-23.2802, -32.5443) (-23.3194, -32.5617) (-23.3586, -32.5794) (-23.3977, -32.5974) (-23.4367, -32.6158) (-23.4757, -32.6345) (-23.5147, -32.6536) (-23.5536, -32.673) (-23.5925, -32.6927) (-23.6313, -32.7128) (-23.67, -32.7331) (-23.7087, -32.7538) (-23.7473, -32.7749) (-23.7859, -32.7962) (-23.8244, -32.8179) (-23.8629, -32.8398) (-23.9013, -32.8621) (-23.9396, -32.8847) (-23.9778, -32.9076) (-24.016, -32.9308) (-24.0541, -32.9543) (-24.0922, -32.9781) (-24.1302, -33.0022) (-24.168, -33.0267) (-24.2059, -33.0514) (-24.2436, -33.0764) (-24.2813, -33.1017) (-24.3188, -33.1273) (-24.3563, -33.1532) (-24.3937, -33.1793) (-24.4236, -33.2005) (-24.446, -33.2165) (-24.4609, -33.2272) (-24.4683, -33.2326) knots 0 0 0 0 0 0 0.01428571 0.02857143 0.04285714 0.05714286 0.07142857 0.08571429 0.1 0.11428571 0.12857143 0.14285714 0.15714286 0.17142857 0.18571429 0.2 0.21428571 0.22857143 0.24285714 0.25714286 0.27142857 0.28571429 0.3 0.31428571 0.32857143 0.34285714 0.35714286 0.37142857 0.38571429 0.4 0.41428571 0.42857143 0.44285714 0.45714286 0.47142857 0.48571429 0.5 0.51428571 0.52857143 0.54285714 0.55714286 0.57142857 0.58571429 0.6 0.61428571 0.62857143 0.64285714 0.65714286 0.67142857 0.68571429 0.7 0.71428571 0.72857143 0.74285714 0.75714286 0.77142857 0.78571429 0.8 0.81428571 0.82857143 0.84285714 0.85714286 0.87142857 0.88571429 0.9 0.91428571 0.92857143 0.94285714 0.95714286 0.97142857 0.98571429 1 1 1 1 1 1
  arc A2 (-24.4683, -33.2326) -> (-24.4683, -34.3177) centre (-12.4806, -33.7751) ccw
  spline S1 degree 5 poles (-24.4683, -34.3177) (-24.4609, -34.3231) (-24.446, -34.3338) (-24.4236, -34.3498) (-24.3937, -34.371) (-24.3563, -34.3971) (-24.3188, -34.423) (-24.2813, -34.4486) (-24.2436, -34.4739) (-24.2059, -34.4989) (-24.168, -34.5236) (-24.1302, -34.548) (-24.0922, -34.5722) (-24.0541, -34.596) (-24.016, -34.6195) (-23.9778, -34.6427) (-23.9396, -34.6656) (-23.9013, -34.6882) (-23.8629, -34.7105) (-23.8244, -34.7324) (-23.7859, -34.7541) (-23.7473, -34.7754) (-23.7087, -34.7964) (-23.67, -34.8171) (-23.6313, -34.8375) (-23.5925, -34.8576) (-23.5536, -34.8773) (-23.5147, -34.8967) (-23.4757, -34.9158) (-23.4367, -34.9345) (-23.3977, -34.9529) (-23.3586, -34.9709) (-23.3194, -34.9886) (-23.2802, -35.006) (-23.241, -35.023) (-23.2017, -35.0397) (-23.1624, -35.056) (-23.1231, -35.0719) (-23.0837, -35.0875) (-23.0443, -35.1027) (-23.0049, -35.1176) (-22.9654, -35.1321) (-22.926, -35.1462) (-22.8865, -35.1599) (-22.847, -35.1732) (-22.8074, -35.1861) (-22.7679, -35.1986) (-22.7283, -35.2108) (-22.6887, -35.2225) (-22.6491, -35.2339) (-22.6095, -35.2448) (-22.5699, -35.2553) (-22.5304, -35.2653) (-22.4908, -35.2748) (-22.4512, -35.2838) (-22.4116, -35.2925) (-22.372, -35.3007) (-22.3325, -35.3085) (-22.2929, -35.3158) (-22.2534, -35.3227) (-22.2139, -35.3289) (-22.1745, -35.3345) (-22.1351, -35.3394) (-22.0957, -35.3435) (-22.0564, -35.347) (-22.0171, -35.35) (-21.9779, -35.3527) (-21.9387, -35.3549) (-21.8996, -35.3567) (-21.8606, -35.3576) (-21.8218, -35.357) (-21.7909, -35.3549) (-21.7678, -35.3522) (-21.7525, -35.3499) (-21.7448, -35.3486) knots -1 -1 -1 -1 -1 -1 -0.98571429 -0.97142857 -0.95714286 -0.94285714 -0.92857143 -0.91428571 -0.9 -0.88571429 -0.87142857 -0.85714286 -0.84285714 -0.82857143 -0.81428571 -0.8 -0.78571429 -0.77142857 -0.75714286 -0.74285714 -0.72857143 -0.71428571 -0.7 -0.68571429 -0.67142857 -0.65714286 -0.64285714 -0.62857143 -0.61428571 -0.6 -0.58571429 -0.57142857 -0.55714286 -0.54285714 -0.52857143 -0.51428571 -0.5 -0.48571429 -0.47142857 -0.45714286 -0.44285714 -0.42857143 -0.41428571 -0.4 -0.38571429 -0.37142857 -0.35714286 -0.34285714 -0.32857143 -0.31428571 -0.3 -0.28571429 -0.27142857 -0.25714286 -0.24285714 -0.22857143 -0.21428571 -0.2 -0.18571429 -0.17142857 -0.15714286 -0.14285714 -0.12857143 -0.11428571 -0.1 -0.08571429 -0.07142857 -0.05714286 -0.04285714 -0.02857143 -0.01428571 0 0 0 0 0 0
  line L1 (-21.7448, -35.3486) -> (-20.4001, -35.1214)
  arc A3 (-19.83, -35.5002) -> (-20.4001, -35.1214) centre (-20.3168, -35.6144) ccw
  arc A4 (-19.83, -35.5002) -> (-19.4404, -36.6995) centre (-12.4806, -33.7751) ccw
  arc A5 (-19.6789, -37.341) -> (-19.4404, -36.6995) centre (-19.9013, -36.8932) ccw
  line L2 (-19.6789, -37.341) -> (-20.9004, -37.9476)
  spline S2 degree 5 poles (-20.9004, -37.9476) (-20.9073, -37.9511) (-20.9211, -37.9582) (-20.9413, -37.9696) (-20.9676, -37.986) (-20.9993, -38.0084) (-21.0304, -38.032) (-21.061, -38.0564) (-21.0913, -38.0813) (-21.1215, -38.1065) (-21.1515, -38.132) (-21.1812, -38.1579) (-21.2107, -38.1844) (-21.2397, -38.2115) (-21.2683, -38.2392) (-21.2966, -38.2675) (-21.3245, -38.2963) (-21.3522, -38.3255) (-21.3796, -38.355) (-21.4068, -38.3849) (-21.4338, -38.4152) (-21.4605, -38.4458) (-21.4869, -38.4767) (-21.513, -38.5081) (-21.5389, -38.5398) (-21.5645, -38.5719) (-21.5899, -38.6044) (-21.615, -38.6372) (-21.6399, -38.6702) (-21.6645, -38.7036) (-21.6889, -38.7373) (-21.713, -38.7713) (-21.7369, -38.8056) (-21.7606, -38.8402) (-21.784, -38.8751) (-21.8072, -38.9103) (-21.8301, -38.9458) (-21.8528, -38.9816) (-21.8752, -39.0176) (-21.8974, -39.0539) (-21.9194, -39.0904) (-21.9411, -39.1272) (-21.9626, -39.1643) (-21.9839, -39.2017) (-22.0049, -39.2392) (-22.0257, -39.2771) (-22.0463, -39.3152) (-22.0666, -39.3535) (-22.0867, -39.392) (-22.1065, -39.4308) (-22.1261, -39.4699) (-22.1455, -39.5091) (-22.1646, -39.5486) (-22.1835, -39.5883) (-22.2022, -39.6283) (-22.2206, -39.6684) (-22.2388, -39.7088) (-22.2568, -39.7494) (-22.2745, -39.7902) (-22.292, -39.8312) (-22.3092, -39.8724) (-22.3263, -39.9139) (-22.343, -39.9555) (-22.3596, -39.9973) (-22.3759, -40.0393) (-22.392, -40.0816) (-22.4078, -40.124) (-22.4234, -40.1666) (-22.4387, -40.2094) (-22.4539, -40.2523) (-22.4687, -40.2955) (-22.4805, -40.3302) (-22.4891, -40.3563) (-22.4949, -40.3737) (-22.4977, -40.3824) knots 0 0 0 0 0 0 0.01428571 0.02857143 0.04285714 0.05714286 0.07142857 0.08571429 0.1 0.11428571 0.12857143 0.14285714 0.15714286 0.17142857 0.18571429 0.2 0.21428571 0.22857143 0.24285714 0.25714286 0.27142857 0.28571429 0.3 0.31428571 0.32857143 0.34285714 0.35714286 0.37142857 0.38571429 0.4 0.41428571 0.42857143 0.44285714 0.45714286 0.47142857 0.48571429 0.5 0.51428571 0.52857143 0.54285714 0.55714286 0.57142857 0.58571429 0.6 0.61428571 0.62857143 0.64285714 0.65714286 0.67142857 0.68571429 0.7 0.71428571 0.72857143 0.74285714 0.75714286 0.77142857 0.78571429 0.8 0.81428571 0.82857143 0.84285714 0.85714286 0.87142857 0.88571429 0.9 0.91428571 0.92857143 0.94285714 0.95714286 0.97142857 0.98571429 1 1 1 1 1 1
  arc A6 (-22.4977, -40.3824) -> (-21.86, -41.2603) centre (-12.4806, -33.7751) ccw
  spline S3 degree 5 poles (-21.86, -41.2603) (-21.8508, -41.2602) (-21.8324, -41.2602) (-21.8049, -41.26) (-21.7683, -41.2596) (-21.7227, -41.2587) (-21.6771, -41.2576) (-21.6317, -41.2563) (-21.5863, -41.2546) (-21.5411, -41.2527) (-21.496, -41.2504) (-21.451, -41.2479) (-21.4061, -41.2451) (-21.3613, -41.242) (-21.3167, -41.2386) (-21.2721, -41.2349) (-21.2277, -41.231) (-21.1834, -41.2267) (-21.1393, -41.2222) (-21.0953, -41.2174) (-21.0514, -41.2122) (-21.0076, -41.2068) (-20.964, -41.2011) (-20.9205, -41.1951) (-20.8772, -41.1888) (-20.834, -41.1823) (-20.791, -41.1754) (-20.7481, -41.1682) (-20.7054, -41.1607) (-20.6628, -41.1529) (-20.6204, -41.1449) (-20.5782, -41.1365) (-20.5361, -41.1278) (-20.4942, -41.1188) (-20.4525, -41.1095) (-20.4109, -41.0999) (-20.3695, -41.09) (-20.3283, -41.0798) (-20.2873, -41.0692) (-20.2465, -41.0584) (-20.2059, -41.0472) (-20.1654, -41.0358) (-20.1252, -41.024) (-20.0852, -41.0118) (-20.0454, -40.9994) (-20.0058, -40.9866) (-19.9665, -40.9735) (-19.9273, -40.9601) (-19.8884, -40.9463) (-19.8497, -40.9322) (-19.8112, -40.9178) (-19.7731, -40.903) (-19.7351, -40.8878) (-19.6975, -40.8722) (-19.6602, -40.8563) (-19.6231, -40.84) (-19.5863, -40.8234) (-19.5497, -40.8064) (-19.5134, -40.7891) (-19.4773, -40.7714) (-19.4417, -40.7533) (-19.4065, -40.7347) (-19.3718, -40.7154) (-19.3375, -40.6956) (-19.3036, -40.6754) (-19.2701, -40.6547) (-19.2368, -40.6338) (-19.2038, -40.6126) (-19.1711, -40.591) (-19.139, -40.5688) (-19.108, -40.5455) (-19.0842, -40.5256) (-19.0671, -40.5099) (-19.0561, -40.499) (-19.0507, -40.4935) knots -1 -1 -1 -1 -1 -1 -0.98571429 -0.97142857 -0.95714286 -0.94285714 -0.92857143 -0.91428571 -0.9 -0.88571429 -0.87142857 -0.85714286 -0.84285714 -0.82857143 -0.81428571 -0.8 -0.78571429 -0.77142857 -0.75714286 -0.74285714 -0.72857143 -0.71428571 -0.7 -0.68571429 -0.67142857 -0.65714286 -0.64285714 -0.62857143 -0.61428571 -0.6 -0.58571429 -0.57142857 -0.55714286 -0.54285714 -0.52857143 -0.51428571 -0.5 -0.48571429 -0.47142857 -0.45714286 -0.44285714 -0.42857143 -0.41428571 -0.4 -0.38571429 -0.37142857 -0.35714286 -0.34285714 -0.32857143 -0.31428571 -0.3 -0.28571429 -0.27142857 -0.25714286 -0.24285714 -0.22857143 -0.21428571 -0.2 -0.18571429 -0.17142857 -0.15714286 -0.14285714 -0.12857143 -0.11428571 -0.1 -0.08571429 -0.07142857 -0.05714286 -0.04285714 -0.02857143 -0.01428571 0 0 0 0 0 0
  line L3 (-19.0507, -40.4935) -> (-18.0963, -39.5193)
  arc A7 (-17.4125, -39.4906) -> (-18.0963, -39.5193) centre (-17.7391, -39.8692) ccw
  arc A8 (-17.4125, -39.4906) -> (-16.3923, -40.2318) centre (-12.4806, -33.7751) ccw
  arc A9 (-16.2082, -40.891) -> (-16.3923, -40.2318) centre (-16.6514, -40.6595) ccw
  line L4 (-16.2082, -40.891) -> (-16.8398, -42.0998)
  spline S4 degree 5 poles (-16.8398, -42.0998) (-16.8434, -42.1066) (-16.8503, -42.1205) (-16.86, -42.1416) (-16.8716, -42.1703) (-16.8842, -42.2071) (-16.8954, -42.2445) (-16.9058, -42.2822) (-16.9157, -42.3202) (-16.9253, -42.3583) (-16.9346, -42.3965) (-16.9434, -42.435) (-16.9517, -42.4737) (-16.9592, -42.5127) (-16.9661, -42.552) (-16.9723, -42.5915) (-16.978, -42.6312) (-16.9832, -42.671) (-16.9881, -42.7111) (-16.9925, -42.7512) (-16.9965, -42.7915) (-17.0001, -42.832) (-17.0033, -42.8726) (-17.006, -42.9133) (-17.0083, -42.9542) (-17.0102, -42.9953) (-17.0116, -43.0364) (-17.0127, -43.0777) (-17.0133, -43.1191) (-17.0136, -43.1606) (-17.0136, -43.2022) (-17.0131, -43.2439) (-17.0123, -43.2857) (-17.0111, -43.3275) (-17.0095, -43.3695) (-17.0076, -43.4116) (-17.0053, -43.4538) (-17.0026, -43.4961) (-16.9996, -43.5384) (-16.9962, -43.5808) (-16.9925, -43.6233) (-16.9884, -43.6659) (-16.984, -43.7085) (-16.9793, -43.7512) (-16.9742, -43.794) (-16.9688, -43.8368) (-16.963, -43.8797) (-16.957, -43.9226) (-16.9505, -43.9656) (-16.9438, -44.0087) (-16.9367, -44.0518) (-16.9293, -44.0949) (-16.9216, -44.1381) (-16.9135, -44.1814) (-16.9051, -44.2247) (-16.8965, -44.268) (-16.8874, -44.3113) (-16.8781, -44.3547) (-16.8685, -44.3982) (-16.8585, -44.4416) (-16.8482, -44.4851) (-16.8377, -44.5286) (-16.8268, -44.5722) (-16.8156, -44.6157) (-16.8041, -44.6593) (-16.7922, -44.7029) (-16.7801, -44.7465) (-16.7677, -44.7902) (-16.755, -44.8338) (-16.7419, -44.8775) (-16.7286, -44.9211) (-16.7177, -44.9561) (-16.7094, -44.9823) (-16.7038, -44.9998) (-16.701, -45.0085) knots 0 0 0 0 0 0 0.01428571 0.02857143 0.04285714 0.05714286 0.07142857 0.08571429 0.1 0.11428571 0.12857143 0.14285714 0.15714286 0.17142857 0.18571429 0.2 0.21428571 0.22857143 0.24285714 0.25714286 0.27142857 0.28571429 0.3 0.31428571 0.32857143 0.34285714 0.35714286 0.37142857 0.38571429 0.4 0.41428571 0.42857143 0.44285714 0.45714286 0.47142857 0.48571429 0.5 0.51428571 0.52857143 0.54285714 0.55714286 0.57142857 0.58571429 0.6 0.61428571 0.62857143 0.64285714 0.65714286 0.67142857 0.68571429 0.7 0.71428571 0.72857143 0.74285714 0.75714286 0.77142857 0.78571429 0.8 0.81428571 0.82857143 0.84285714 0.85714286 0.87142857 0.88571429 0.9 0.91428571 0.92857143 0.94285714 0.95714286 0.97142857 0.98571429 1 1 1 1 1 1
  arc A10 (-16.701, -45.0085) -> (-15.669, -45.3438) centre (-12.4806, -33.7751) ccw
  spline S5 degree 5 poles (-15.669, -45.3438) (-15.6616, -45.3384) (-15.6468, -45.3275) (-15.6246, -45.3112) (-15.5953, -45.2894) (-15.5588, -45.2619) (-15.5226, -45.2342) (-15.4867, -45.2064) (-15.451, -45.1784) (-15.4155, -45.1502) (-15.3803, -45.1219) (-15.3454, -45.0934) (-15.3107, -45.0647) (-15.2763, -45.0359) (-15.2422, -45.0069) (-15.2083, -44.9778) (-15.1747, -44.9485) (-15.1414, -44.919) (-15.1084, -44.8894) (-15.0756, -44.8596) (-15.0431, -44.8297) (-15.0109, -44.7996) (-14.9789, -44.7693) (-14.9473, -44.7389) (-14.9159, -44.7084) (-14.8849, -44.6777) (-14.8541, -44.6468) (-14.8236, -44.6158) (-14.7935, -44.5846) (-14.7636, -44.5533) (-14.734, -44.5219) (-14.7048, -44.4902) (-14.6759, -44.4585) (-14.6472, -44.4266) (-14.6189, -44.3945) (-14.591, -44.3623) (-14.5633, -44.33) (-14.536, -44.2975) (-14.509, -44.2649) (-14.4823, -44.2321) (-14.456, -44.1992) (-14.4301, -44.1662) (-14.4045, -44.133) (-14.3792, -44.0996) (-14.3544, -44.0662) (-14.3298, -44.0326) (-14.3057, -43.9988) (-14.2819, -43.965) (-14.2585, -43.9309) (-14.2355, -43.8968) (-14.2129, -43.8625) (-14.1907, -43.8281) (-14.1689, -43.7935) (-14.1476, -43.7588) (-14.1268, -43.724) (-14.1064, -43.689) (-14.0863, -43.6539) (-14.0667, -43.6187) (-14.0475, -43.5833) (-14.0288, -43.5479) (-14.0106, -43.5123) (-13.9931, -43.4765) (-13.9763, -43.4405) (-13.9602, -43.4043) (-13.9447, -43.368) (-13.9297, -43.3316) (-13.9151, -43.2951) (-13.9008, -43.2586) (-13.887, -43.2219) (-13.8742, -43.1851) (-13.8627, -43.148) (-13.8552, -43.1179) (-13.8506, -43.0952) (-13.8481, -43.0799) (-13.847, -43.0722) knots -1 -1 -1 -1 -1 -1 -0.98571429 -0.97142857 -0.95714286 -0.94285714 -0.92857143 -0.91428571 -0.9 -0.88571429 -0.87142857 -0.85714286 -0.84285714 -0.82857143 -0.81428571 -0.8 -0.78571429 -0.77142857 -0.75714286 -0.74285714 -0.72857143 -0.71428571 -0.7 -0.68571429 -0.67142857 -0.65714286 -0.64285714 -0.62857143 -0.61428571 -0.6 -0.58571429 -0.57142857 -0.55714286 -0.54285714 -0.52857143 -0.51428571 -0.5 -0.48571429 -0.47142857 -0.45714286 -0.44285714 -0.42857143 -0.41428571 -0.4 -0.38571429 -0.37142857 -0.35714286 -0.34285714 -0.32857143 -0.31428571 -0.3 -0.28571429 -0.27142857 -0.25714286 -0.24285714 -0.22857143 -0.21428571 -0.2 -0.18571429 -0.17142857 -0.15714286 -0.14285714 -0.12857143 -0.11428571 -0.1 -0.08571429 -0.07142857 -0.05714286 -0.04285714 -0.02857143 -0.01428571 0 0 0 0 0 0
  line L5 (-13.847, -43.0722) -> (-13.6474, -41.7231)
  arc A11 (-13.1111, -41.298) -> (-13.6474, -41.7231) centre (-13.1528, -41.7962) ccw
  arc A12 (-13.1111, -41.298) -> (-11.8501, -41.298) centre (-12.4806, -33.7751) ccw
  arc A13 (-11.3137, -41.7231) -> (-11.8501, -41.298) centre (-11.8083, -41.7962) ccw
  line L6 (-11.3137, -41.7231) -> (-11.1142, -43.0722)
  spline S6 degree 5 poles (-11.1142, -43.0722) (-11.113, -43.0799) (-11.1105, -43.0952) (-11.106, -43.1179) (-11.0984, -43.148) (-11.087, -43.1851) (-11.0741, -43.2219) (-11.0603, -43.2586) (-11.046, -43.2951) (-11.0314, -43.3316) (-11.0164, -43.368) (-11.001, -43.4043) (-10.9849, -43.4405) (-10.9681, -43.4765) (-10.9505, -43.5123) (-10.9324, -43.5479) (-10.9136, -43.5833) (-10.8944, -43.6187) (-10.8748, -43.6539) (-10.8548, -43.689) (-10.8343, -43.724) (-10.8135, -43.7588) (-10.7922, -43.7935) (-10.7705, -43.8281) (-10.7483, -43.8625) (-10.7257, -43.8968) (-10.7026, -43.9309) (-10.6792, -43.965) (-10.6554, -43.9988) (-10.6313, -44.0326) (-10.6068, -44.0662) (-10.5819, -44.0996) (-10.5567, -44.133) (-10.5311, -44.1662) (-10.5051, -44.1992) (-10.4788, -44.2321) (-10.4521, -44.2649) (-10.4251, -44.2975) (-10.3978, -44.33) (-10.3702, -44.3623) (-10.3422, -44.3945) (-10.3139, -44.4266) (-10.2853, -44.4585) (-10.2563, -44.4902) (-10.2271, -44.5219) (-10.1975, -44.5533) (-10.1677, -44.5846) (-10.1375, -44.6158) (-10.107, -44.6468) (-10.0763, -44.6777) (-10.0452, -44.7084) (-10.0138, -44.7389) (-9.9822, -44.7693) (-9.9503, -44.7996) (-9.9181, -44.8297) (-9.8856, -44.8596) (-9.8528, -44.8894) (-9.8197, -44.919) (-9.7864, -44.9485) (-9.7528, -44.9778) (-9.7189, -45.0069) (-9.6848, -45.0359) (-9.6504, -45.0647) (-9.6157, -45.0934) (-9.5808, -45.1219) (-9.5456, -45.1502) (-9.5102, -45.1784) (-9.4745, -45.2064) (-9.4385, -45.2342) (-9.4023, -45.2619) (-9.3658, -45.2894) (-9.3365, -45.3112) (-9.3144, -45.3275) (-9.2995, -45.3384) (-9.2921, -45.3438) knots 0 0 0 0 0 0 0.01428571 0.02857143 0.04285714 0.05714286 0.07142857 0.08571429 0.1 0.11428571 0.12857143 0.14285714 0.15714286 0.17142857 0.18571429 0.2 0.21428571 0.22857143 0.24285714 0.25714286 0.27142857 0.28571429 0.3 0.31428571 0.32857143 0.34285714 0.35714286 0.37142857 0.38571429 0.4 0.41428571 0.42857143 0.44285714 0.45714286 0.47142857 0.48571429 0.5 0.51428571 0.52857143 0.54285714 0.55714286 0.57142857 0.58571429 0.6 0.61428571 0.62857143 0.64285714 0.65714286 0.67142857 0.68571429 0.7 0.71428571 0.72857143 0.74285714 0.75714286 0.77142857 0.78571429 0.8 0.81428571 0.82857143 0.84285714 0.85714286 0.87142857 0.88571429 0.9 0.91428571 0.92857143 0.94285714 0.95714286 0.97142857 0.98571429 1 1 1 1 1 1
  arc A14 (-9.2921, -45.3438) -> (-8.2602, -45.0085) centre (-12.4806, -33.7751) ccw